Autodesk Fusion 360 part; units mm, degrees
(part 2 of 2)
sketch "Sketch6" plane through (0, 0, 0.5) normal (0, 0, -1) x (1, 0, 0)
  line L0 (106.2459, 65.5638) -> (-30.2459, 65.5638)
  arc A0 (-30.2459, 65.5638) -> (-39.5638, 56.2459) centre (-30.2459, 56.2459) ccw
  line L1 (-39.5638, 56.2459) -> (-39.5638, -30.2459)
  arc A1 (-39.5638, -30.2459) -> (-30.2459, -39.5638) centre (-30.2459, -30.2459) ccw
  line L2 (-30.2459, -39.5638) -> (106.2459, -39.5638)
  arc A2 (106.2459, -39.5638) -> (115.5638, -30.2459) centre (106.2459, -30.2459) ccw
  line L3 (115.5638, -30.2459) -> (115.5638, 56.2459)
  arc A3 (115.5638, 56.2459) -> (106.2459, 65.5638) centre (106.2459, 56.2459) ccw
  line L4 (38, 65.5638) -> (38, -39.5638) construction
  line L5 (-39.5638, 13) -> (115.5638, 13) construction
  line L6 (92, -25.5) -> (-16, -25.5)
  line L7 (-20, -21.5) -> (-20, 47.5)
  line L8 (-16, 51.5) -> (92, 51.5)
  line L9 (96, 47.5) -> (96, -21.5)
  line L10 (96, -25.5) -> (-20, 51.5) construction
  line L11 (-20, -25.5) -> (96, 51.5) construction
  arc A4 (-16, 51.5) -> (-20, 47.5) centre (-16, 47.5) ccw
  arc A5 (96, 47.5) -> (92, 51.5) centre (92, 47.5) ccw
  arc A6 (92, -25.5) -> (96, -21.5) centre (92, -21.5) ccw
  arc A7 (-20, -21.5) -> (-16, -25.5) centre (-16, -21.5) ccw
  point P0 (38, 13)
  dimension "d58" = 116
  dimension "d59" = 77
  dimension "d68" = 4
  dimension "d69" = 4
  dimension "d70" = 4
  dimension "d71" = 4
  constraint midpoint L0 L4.start
  constraint midpoint L2 L4.end
  constraint midpoint L1 L5.start
  constraint midpoint L3 L5.end
  constraint horizontal L6
  constraint perpendicular L6 L7
  constraint parallel L6 L8
  constraint parallel L7 L9
  constraint coincident L10 P0
  constraint coincident L11 P0
  constraint midpoint L5 P0
  constraint coincident L10.end L8
  constraint coincident L10.end L7
  constraint tangent L8 A4
  constraint tangent L7 A4
  constraint coincident L11.end L8
  constraint coincident L11.end L9
  constraint tangent L8 A5
  constraint tangent L9 A5
  constraint coincident L10.start L9
  constraint coincident L10.start L6
  constraint tangent L9 A6
  constraint tangent L6 A6
  constraint coincident L11.start L7
  constraint coincident L11.start L6
  constraint tangent L7 A7
  constraint tangent L6 A7
  measures "d58" distance of L10.end L11.end
  measures "d59" distance of L11.start L10.end
  measures "d68" radius of A4
  measures "d69" radius of A5
  measures "d70" radius of A6
  measures "d71" radius of A7
extrude "Extrude8" cut sketch "Sketch6" against normal blind 1.1 contours L6 L7 L8 L9 A4 A5 A6 A7
sketch "Sketch7" plane through (0, 0, 1.6) normal (0, 0, -1) x (1, 0, 0)
  line L0 (92, 51.5) -> (-16, 51.5)
  line L1 (-20, 47.5) -> (-20, -21.5)
  line L2 (-16, -25.5) -> (92, -25.5)
  line L3 (96, -21.5) -> (96, 47.5)
  line L4 (38, 51.5) -> (38, -25.5) construction
  line L5 (96, 13) -> (-20, 13) construction
  line L6 (87, -20.5) -> (-11, -20.5)
  line L7 (-15, -16.5) -> (-15, 42.5)
  line L8 (-11, 46.5) -> (87, 46.5)
  line L9 (91, 42.5) -> (91, -16.5)
  line L10 (91, -20.5) -> (-15, 46.5) construction
  line L11 (-15, -20.5) -> (91, 46.5) construction
  arc A0 (-16, 51.5) -> (-20, 47.5) centre (-16, 47.5) ccw
  arc A1 (-20, -21.5) -> (-16, -25.5) centre (-16, -21.5) ccw
  arc A2 (92, -25.5) -> (96, -21.5) centre (92, -21.5) ccw
  arc A3 (96, 47.5) -> (92, 51.5) centre (92, 47.5) ccw
  arc A4 (-11, 46.5) -> (-15, 42.5) centre (-11, 42.5) ccw
  arc A5 (91, 42.5) -> (87, 46.5) centre (87, 42.5) ccw
  arc A6 (87, -20.5) -> (91, -16.5) centre (87, -16.5) ccw
  arc A7 (-15, -16.5) -> (-11, -20.5) centre (-11, -16.5) ccw
  point P0 (38, 13)
  dimension "d62" = 106
  dimension "d65" = 67
  dimension "d72" = 4
  dimension "d73" = 4
  dimension "d74" = 4
  dimension "d75" = 4
  constraint midpoint L0 L4.start
  constraint midpoint L2 L4.end
  constraint midpoint L3 L5.start
  constraint midpoint L1 L5.end
  constraint horizontal L6
  constraint perpendicular L6 L7
  constraint parallel L6 L8
  constraint parallel L7 L9
  constraint coincident L10 P0
  constraint coincident L11 P0
  constraint midpoint L4 P0
  constraint coincident L10.end L8
  constraint coincident L10.end L7
  constraint tangent L8 A4
  constraint tangent L7 A4
  constraint coincident L11.end L9
  constraint coincident L11.end L8
  constraint tangent L9 A5
  constraint tangent L8 A5
  constraint coincident L10.start L9
  constraint coincident L10.start L6
  constraint tangent L9 A6
  constraint tangent L6 A6
  constraint coincident L11.start L6
  constraint coincident L11.start L7
  constraint tangent L6 A7
  constraint tangent L7 A7
  measures "d62" distance of L10.end L11.end
  measures "d65" distance of L11.start L10.end
  measures "d72" radius of A4
  measures "d73" radius of A5
  measures "d74" radius of A6
  measures "d75" radius of A7
extrude "Extrude9" cut sketch "Sketch7" against normal blind 8.4 contours L6 L7 L8 L9 A4 A5 A6 A7
sketch "Sketch9" plane through (0, 0, 6) normal (0, 0, 1) x (-1, 0, 0)
  line L0 (15, 42.5) -> (15, -16.5)
  arc A0 (11, -20.5) -> (15, -16.5) centre (11, -16.5) ccw
  line L1 (11, -20.5) -> (-87, -20.5)
  arc A1 (-91, -16.5) -> (-87, -20.5) centre (-87, -16.5) ccw
  line L2 (-91, -16.5) -> (-91, 42.5)
  arc A2 (-87, 46.5) -> (-91, 42.5) centre (-87, 42.5) ccw
  line L3 (-87, 46.5) -> (11, 46.5)
  arc A3 (15, 42.5) -> (11, 46.5) centre (11, 42.5) ccw
  circle A4 centre (-121, 71) radius 2
  circle A5 centre (-121, -45) radius 2
  circle A6 centre (45, 71) radius 2
  circle A7 centre (45, -45) radius 2
  arc A8 (48, -52) -> (52, -48) centre (48, -48) ccw
  line L4 (52, -48) -> (52, 74)
  arc A9 (52, 74) -> (48, 78) centre (48, 74) ccw
  line L5 (48, 78) -> (-124, 78)
  arc A10 (-124, 78) -> (-128, 74) centre (-124, 74) ccw
  line L6 (-128, 74) -> (-128, -48)
  arc A11 (-128, -48) -> (-124, -52) centre (-124, -48) ccw
  line L7 (-124, -52) -> (48, -52)
  line L8 (45, -47) -> (45, -43) construction
  line L9 (43, -45) -> (47, -45) construction
  circle A12 centre (45, -45) radius 4.11
  line L10 (-38, -52) -> (-38, 78) construction
  line L11 (-128, 13) -> (52, 13) construction
  circle A13 centre (-121, -45) radius 4.11
  circle A14 centre (45, 71) radius 4.11
  circle A15 centre (-121, 71) radius 4.11
  dimension "d91" = 8.22
  constraint coincident A7 L8.start
  constraint coincident A7 L8.end
  constraint vertical L8
  constraint coincident A7 L9.start
  constraint coincident A7 L9.end
  constraint perpendicular L8 L9
  constraint concentric A7 A12
  constraint midpoint L7 L10.start
  constraint midpoint L5 L10.end
  constraint midpoint L6 L11.start
  constraint midpoint L4 L11.end
  constraint symmetric A12 L10 A13
  constraint symmetric A12 L11 A14
  constraint symmetric L11 A13 A15
  measures "d91" diameter of A12
extrude "Extrude11" cut sketch "Sketch9" against normal blind 4 contours A12 | A13 | A14 | A15
sketch "Sketch10" plane through (0, 0, 0.5) normal (0, 0, -1) x (1, 0, 0)
  line L0 (-20, -21.5) -> (-20, 47.5)
  arc A0 (-16, 51.5) -> (-20, 47.5) centre (-16, 47.5) ccw
  line L1 (-16, 51.5) -> (92, 51.5)
  arc A1 (96, 47.5) -> (92, 51.5) centre (92, 47.5) ccw
  line L2 (96, 47.5) -> (96, -21.5)
  arc A2 (92, -25.5) -> (96, -21.5) centre (92, -21.5) ccw
  line L3 (92, -25.5) -> (-16, -25.5)
  arc A3 (-20, -21.5) -> (-16, -25.5) centre (-16, -21.5) ccw
  line L4 (106.2459, 65.5638) -> (-30.2459, 65.5638)
  arc A4 (-30.2459, 65.5638) -> (-39.5638, 56.2459) centre (-30.2459, 56.2459) ccw
  line L5 (-39.5638, 56.2459) -> (-39.5638, -30.2459)
  arc A5 (-39.5638, -30.2459) -> (-30.2459, -39.5638) centre (-30.2459, -30.2459) ccw
  line L6 (-30.2459, -39.5638) -> (106.2459, -39.5638)
  arc A6 (106.2459, -39.5638) -> (115.5638, -30.2459) centre (106.2459, -30.2459) ccw
  line L7 (115.5638, -30.2459) -> (115.5638, 56.2459)
  arc A7 (115.5638, 56.2459) -> (106.2459, 65.5638) centre (106.2459, 56.2459) ccw
  line L8 (38, 65.5638) -> (38, -39.5638) construction
  line L9 (115.5638, 13) -> (-39.5638, 13) construction
  line L10 (38, 13) -> (-24.24, 13) construction
  line L11 (-23.09, 11) -> (-25.39, 11)
  line L12 (-25.39, 11) -> (-25.39, 15)
  line L13 (-25.39, 15) -> (-23.09, 15)
  line L14 (-23.09, 15) -> (-23.09, 11)
  line L15 (-23.09, 11) -> (-25.39, 15) construction
  line L16 (-25.39, 11) -> (-23.09, 15) construction
  line L17 (38, 13) -> (38, 54) construction
  line L18 (40, 52.85) -> (36, 52.85)
  line L19 (36, 52.85) -> (36, 55.15)
  line L20 (36, 55.15) -> (40, 55.15)
  line L21 (40, 55.15) -> (40, 52.85)
  line L22 (40, 52.85) -> (36, 55.15) construction
  line L23 (36, 52.85) -> (40, 55.15) construction
  line L24 (99.09, 15) -> (99.09, 11)
  line L25 (101.39, 15) -> (99.09, 15)
  line L26 (101.39, 11) -> (101.39, 15)
  line L27 (99.09, 11) -> (101.39, 11)
  line L28 (40, -26.85) -> (36, -26.85)
  line L29 (40, -29.15) -> (40, -26.85)
  line L30 (36, -29.15) -> (40, -29.15)
  line L31 (36, -26.85) -> (36, -29.15)
  point P0 (-24.24, 13)
  point P1 (38, 54)
  dimension "d97" = 62.24
  dimension "d98" = 2.3
  dimension "d99" = 4
  dimension "d100" = 41
  dimension "d101" = 2.3
  dimension "d102" = 4
  constraint midpoint L4 L8.start
  constraint midpoint L6 L8.end
  constraint midpoint L7 L9.start
  constraint midpoint L5 L9.end
  constraint midpoint L9 L10.start
  constraint perpendicular L8 L10
  constraint horizontal L11
  constraint perpendicular L11 L12
  constraint parallel L11 L13
  constraint parallel L12 L14
  constraint coincident L15 P0
  constraint coincident L16 P0
  constraint coincident P0 L10.end
  constraint perpendicular L9 L17
  constraint horizontal L18
  constraint perpendicular L18 L19
  constraint parallel L18 L20
  constraint parallel L19 L21
  constraint coincident L22 P1
  constraint coincident L23 P1
  constraint coincident P1 L17.end
  constraint symmetric L8 L11.start L24.end
  constraint symmetric L8 L11.end L26.start
  constraint symmetric L8 L12.end L25.start
  constraint symmetric L8 L13.end L24.start
  constraint symmetric L9 L18.start L28.start
  constraint symmetric L9 L18.end L28.end
  constraint symmetric L9 L19.end L30.start
  constraint symmetric L9 L20.end L29.start
  measures "d97" distance of L10.start P0
  measures "d98" distance of L12.end L13.end
  measures "d99" distance of L11.end L12.end
  measures "d100" distance of L10.start P1
  measures "d101" distance of L18.start L20.end
  measures "d102" distance of L19.end L20.end
extrude "Extrude12" add sketch "Sketch10" along normal blind 4.2 contours L11 L12 L13 L14 | L18 L19 L20 L21 | L24 L25 L26 L27 | L28 L29 L30 L31
chamfer "Chamfer1" distance 0.5 angle 45 4 edges at (-41.1681, 43.5138, 6) (124.8319, 43.5138, 6) (124.8319, -72.4862, 6) (-41.1681, -72.4862, 6)
equation "d3 = Bolt_Diam"
equation "ORingDiameter = 1.78 mm" comment "Diamter of the O ring"
equation "ORingInnerDiameter = 170 mm" comment "Inner diamter of the o ring bore"
equation "d25 = ( ORingPerimeter - 100 mm ) / 4 + 50 mm"
equation "ORingPerimeter = 2 * 3.1412 * ( ( ORingInnerDiameter / 2 ) + ORingDiameter / 2 )"
equation "d27 = ( ORingPerimeter - 100 mm ) / 4"
equation "d28 = ( ( ORingDiameter * 1.05 ) / 2 ) + 1.2 mm"
equation "d29 = ( ( ORingDiameter * 1.05 ) / 2 ) + 1.2 mm"
equation "d30 = ( ( ORingDiameter * 1.05 ) / 2 ) + 1.2 mm"
equation "d31 = ( ( ORingDiameter * 1.05 ) / 2 ) + 1.2 mm"
equation "d32 = ORingDiameter * 0.8"
equation "d36 = ( ORingPerimeter - 100 mm ) / 4 + 50 mm"
equation "d37 = ( ORingPerimeter - 100 mm ) / 4"
equation "d38 = ( ORingDiameter * 1.05 ) / 2"
equation "d39 = ( ORingDiameter * 1.05 ) / 2"
equation "d40 = ( ORingDiameter * 1.05 ) / 2"
equation "d41 = ( ORingDiameter * 1.05 ) / 2"
equation "d44 = ( ORingDiameter ) * 6 + ORingDiameter * 0.05 - 1.2 mm"
equation "d45 = ( ORingDiameter ) * 6 + ( ORingDiameter * 1.1 ) + 1.2 mm"
equation "d50 = ( ORingDiameter ) * 6 + ORingDiameter * 0.05 - 0.0 mm"
equation "d51 = ( ORingDiameter ) * 6 + ORingDiameter * 1.1 + 0 mm"
equation "d52 = -( ORingDiameter * 0.8 )"
equation "PanelWidth = 77 mm"
equation "PanelLength = 116 mm"
equation "d58 = PanelLength"
equation "d59 = PanelWidth"
equation "d62 = PanelLength - 10 mm"
equation "d65 = PanelWidth - 10 mm"
equation "d91 = Bolt_Head_Diam + 1 mm"
equation "Bolt_Diam = 4 mm" comment "Diameter of the bolt"
equation "Bolt_Head_Height = 4 mm" comment "Height of th ebolt head"
equation "Bolt_Head_Diam = 7.22 mm" comment "Diamter of the bolt head"
equation "d95 = -Bolt_Head_Height"
